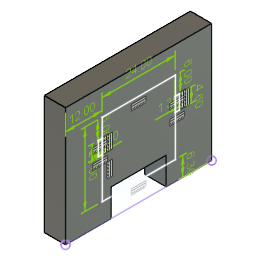
Cameramount2 (Autodesk Fusion 360 design; units mm, degrees)
part number: 2026-05-11-20-39-44-595
Autodesk Fusion 360 part; units mm, degrees
note: some values were not read from the file. Chosen so that the rebuilt part matches the saved one: which bodies a step acts on.
sketch "Sketch1" plane through (0, 0, 0) normal (0, 0, 1) x (1, 0, 0)
  line L0 (0, 0) -> (7, 0)
  line L1 (7, 0) -> (7, 48)
  line L2 (7, 48) -> (0, 48)
  line L3 (0, 48) -> (0, 0)
  circle A0 centre (3.5, 40.5) radius 1.35
  circle A1 centre (3.5, 7.5) radius 1.35
  line L4 (0, 33) -> (7, 33)
  line L5 (0, 15) -> (7, 15)
  dimension "d1" = 7
  dimension "d2" = 48
  dimension "d3" = 2.7
  dimension "d4" = 2.7
  dimension "d5" = 3.5
  dimension "d6" = 3.5
  dimension "d7" = 33
  dimension "d8" = 7.5
  dimension "d9" = 15
  dimension "d10" = 15
  constraint horizontal L0
  constraint vertical L1
  constraint horizontal L2
  constraint vertical L3
  constraint coincident L0.start L3.end
  constraint coincident L3 L4.start
  constraint coincident L1 L4.end
  constraint perpendicular L1 L4
  constraint coincident L3 L5.start
  constraint coincident L1 L5.end
  constraint perpendicular L1 L5
  measures "d1" distance of L0.start L0.end
  measures "d2" distance of L0.start L2.end
  measures "d3" diameter of A0
  measures "d4" diameter of A1
  measures "d5" distance of L3 A0.centre
  measures "d6" distance of L3 A1.centre
  measures "d7" distance of A0.centre A1.centre
  measures "d8" distance of L2 A0.centre
  measures "d9" distance of L2 L4
  measures "d10" distance of L0 L5
extrude "Extrude1" add sketch "Sketch1" along normal blind 13 contours L0 L1 L3 L5 | L1 L2 L3 L4 makes body 1 at (0, 43, 4.3333) makes body 2 at (0, 10, 4.3333)
extrude "Extrude2" add sketch "Sketch1" along normal blind 30 from surface at 9 contours L0 L1 L3 L5 | L1 L3 L4 L5 | L1 L2 L3 L4 | A0 | A1 bodies 1 2
sketch "Sketch2" plane through (7, 0, 0) normal (1, 0, 0) x (0, 1, 0)
  line L0 (33, 0) -> (48, 0)
  line L1 (48, 0) -> (48, 39)
  line L2 (48, 39) -> (0, 39)
  line L3 (0, 39) -> (0, 0)
  line L4 (0, 0) -> (15, 0)
  line L5 (15, 0) -> (15, 9)
  line L6 (15, 9) -> (33, 9)
  line L7 (33, 9) -> (33, 0)
  line L8 (12, 30.3) -> (36, 30.3)
  line L9 (36, 30.3) -> (36, 6.3)
  line L10 (36, 6.3) -> (12, 6.3)
  line L11 (12, 6.3) -> (12, 30.3)
  line L12 (0, 0) -> (48, 0)
  line L13 (12, 24.3) -> (10.7, 24.3)
  line L14 (10.7, 24.3) -> (10.7, 19.7)
  line L15 (10.7, 19.7) -> (12, 19.7)
  line L16 (12, 19.7) -> (12, 24.3)
  line L17 (36, 24.3) -> (37.3, 24.3)
  line L18 (37.3, 24.3) -> (37.3, 19.7)
  line L19 (37.3, 19.7) -> (36, 19.7)
  line L20 (36, 19.7) -> (36, 24.3)
  dimension "d18" = 24
  dimension "d19" = 24
  dimension "d20" = 12
  dimension "d22" = 6.3
  dimension "d31" = 6
  dimension "d32" = 6
  dimension "d33" = 4.6
  dimension "d34" = 4.6
  dimension "d35" = 1.3
  dimension "d36" = 1.3
  constraint horizontal L8
  constraint vertical L9
  constraint horizontal L10
  constraint vertical L11
  constraint horizontal L13
  constraint vertical L14
  constraint horizontal L15
  constraint vertical L16
  constraint coincident L11 L13.start
  constraint horizontal L17
  constraint vertical L18
  constraint horizontal L19
  constraint vertical L20
  constraint coincident L9 L17.start
  measures "d18" distance of L8.start L8.end
  measures "d19" distance of L8.start L10.end
  measures "d20" distance of L3 L11
  measures "d22" distance of L10 L12
  measures "d31" distance of L8 L13
  measures "d32" distance of L8 L17
  measures "d33" distance of L13.end L14.end
  measures "d34" distance of L17.end L18.end
  measures "d35" distance of L9 L18
  measures "d36" distance of L11 L14
extrude "Extrude3" [rolled back] along distance -7 taper angle 0
fillet "Fillet3" [rolled back] radius 5
sketch "Sketch3" plane through (0, 48, 0) normal (0, 1, 0) x (-1, 0, 0)
  line L0 (-2, 39) -> (-2, 0)
  line L1 (-2, 0) -> (0, 0)
  line L2 (0, 0) -> (0, 39)
  line L3 (0, 0) -> (-7.1424, 2)
  line L4 (-7.1424, 2) -> (-7.1424, 0)
  line L5 (-7.1424, 0) -> (0, 0)
  line L6 (0, 39) -> (-2, 39)
  dimension "d39" = 2
  constraint coincident L1.end L2.start
  constraint parallel L0 L4
  constraint perpendicular L4 L5
  measures "d39" distance of L3.end L4.end
fillet "Fillet4" [rolled back] radius 7
extrude "Extrude4" [rolled back] along distance -50 taper angle 0
fillet "Fillet2" [suppressed]
equation "d14 = 28.00 mm + 2 mm"
